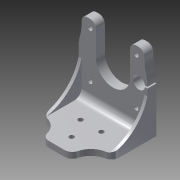
# Autodesk Inventor part: bottom-right bracket
Saved by Autodesk Inventor 2015 SP1 (Build 190203100, 203)
## iProperties
Created: 2015-01-03
Part Number: bottom-right bracket
Material: ABS Plastic
Document SubType Name: Modeling
Designer: Luna
Density: 1.06 g/cm^3
Appearance: Smooth - White
Mass: 2.06395 g
Surface Area: 14.6209 cm^2
Volume: 1.94712 cm^3
Author: Luna
Autodesk Inventor part; units mm, degrees
ref_plane "YZ Plane" through (0, 0, 0) normal (1, 0, 0) x (0, 1, 0)
ref_plane "XZ Plane" through (0, 0, 0) normal (0, 1, 0) x (-1, 0, 0)
ref_plane "XY Plane" through (0, 0, 0) normal (0, 0, 1) x (1, 0, 0)
sketch "hole points" plane through (0, 0, 0) normal (0, 0, 1) x (1, 0, 0)
  line L0 (-7, 0) -> (7, 0) construction
  line L1 (0, 0) -> (0, -13) construction
  dimension "d0" = 14
  dimension "d1" = 13
  constraints: 4 coincident, 4 end point, 1 horizontal, 1 midpoint, 1 vertical
  measures "d0" distance of L0.start L0.end
  measures "d1" distance of L1.start L1.end
sketch "Sketch3" plane through (0, 0, 0) normal (0, 0, 1) x (1, 0, 0)
  line L0 (-7, 0) -> (7, 0) construction
  line L1 (-7, 0) -> (7, 0) construction
  line L2 (-9, -2) -> (9, -2)
  line L3 (9, -2) -> (9, 2)
  line L4 (9, 2) -> (-9, 2)
  line L5 (-9, 2) -> (-9, -2)
  line L6 (-9, -2) -> (9, 2) construction
  line L7 (9, -2) -> (-9, 2) construction
  line L8 (0, 0) -> (0, -13) construction
  line L9 (-2, 2) -> (2, 2)
  line L10 (2, 2) -> (2, -15)
  line L11 (2, -15) -> (-2, -15)
  line L12 (-2, -15) -> (-2, 2)
  line L13 (17, -10) -> (-17, -10)
  line L14 (-17, -10) -> (-17, 10)
  line L15 (-17, 10) -> (17, 10)
  line L16 (17, 10) -> (17, -10)
  line L17 (10, -23) -> (10, 10)
  line L18 (10, 10) -> (-10, 10)
  line L19 (-10, 10) -> (-10, -23)
  line L20 (-10, -23) -> (10, -23)
  point P0 (0, -6.5)
  point P1 (0, 2)
  point P2 (0, -6.5)
  point P3 (0, 2)
  dimension "d31" = 18
  dimension "d32" = 4
  dimension "d33" = 4
  dimension "d34" = 17
  dimension "d35" = 8
  dimension "d36" = 8
  constraints: 40 end point, 8 parallel, 6 midpoint, 4 perpendicular, 2 horizontal, 1 coincident, 1 vertical alignment, 6 other
  measures "d31" distance of L4.end L3.end
  measures "d32" distance of L3.end L2.end
  measures "d33" distance of L10.end L11.end
  measures "d34" distance of L9.end L10.end
  measures "d35" distance between parallel lines of L2 L13
  measures "d36" distance between parallel lines of L10 L17
extrude "back plate Extrusion2" add sketch "Sketch3" against normal blind 4
hole "Hole3" at (-7, 0, 0) at (7, 0, 0) at (0, -13, 0) direction (0, 0, -1) diameter 3.2 end through all
sketch "Sketch4" plane through (-17, 10, 0) normal (0, 1, 0) x (1, 0, 0)
  circle A0 centre (17.85, -27.15) radius 11 projected
  circle A1 centre (2.35, -42.65) radius 1.5 projected
  circle A2 centre (33.35, -11.65) radius 1.5 projected
  circle A3 centre (33.35, -42.65) radius 1.5 projected
  circle A4 centre (2.35, -11.65) radius 1.5 projected
  line L0 (-3.3, -10) -> (0.7, -6) projected
  line L1 (-3.3, -44.3) -> (-3.3, -10) projected
  line L2 (0.7, -48.3) -> (-3.3, -44.3) projected
  line L3 (35, -48.3) -> (0.7, -48.3) projected
  line L4 (39, -44.3) -> (35, -48.3) projected
  line L5 (39, -10) -> (39, -44.3) projected
  line L6 (35, -6) -> (39, -10) projected
  line L7 (0.7, -6) -> (35, -6) projected
  line L8 (-3.3, 0) -> (39, 0)
  line L9 (39, 0) -> (39, 4)
  line L10 (39, 4) -> (-3.3, 4)
  line L11 (-3.3, 4) -> (-3.3, 0)
  line L12 (0, 4) -> (34, 4) projected
  point P0 (17, 0)
  point P1 (17.85, 4)
  point P2 (17, 4)
  point P3 (-3.3, 2)
  point P4 (39, 2)
  dimension "d44" = 4
  constraints: 8 end point, 4 midpoint, 2 parallel, 2 vertical alignment, 1 horizontal, 1 horizontal alignment, 1 perpendicular
  measures "d44" distance of L9.end L8.end
extrude "Extrusion3" add sketch "Sketch4" along normal blind 10 contours L11 L10 L9 L8
sketch "Sketch5" plane through (0, 0, 0) normal (0, 0, 1) x (1, 0, 0)
  line L0 (-16.3, 14) -> (18, 14) projected
  line L1 (-20.3, 20) -> (22, 20)
  line L2 (22, 20) -> (22, 14)
  line L3 (22, 14) -> (-20.3, 14)
  line L4 (-20.3, 14) -> (-20.3, 20)
  point P0 (0, 0)
  dimension "d47" = 42.3
  constraints: 8 end point, 2 parallel, 1 horizontal, 1 perpendicular, 1 point on line
  measures "d47" distance between parallel lines of L2 L4
extrude "Extrusion4" add sketch "Sketch5" along normal blind 48
sketch "Sketch6" plane through (-17, 20, 0) normal (0, 1, 0) x (1, 0, 0)
  circle A0 centre (17.85, -27.15) radius 10.5 projected
  circle A1 centre (17.85, -27.15) radius 11.5
  circle A2 centre (2.35, -42.65) radius 1.5 construction
  circle A3 centre (33.35, -42.65) radius 1.5 construction
  circle A4 centre (33.35, -11.65) radius 1.5 construction
  circle A5 centre (2.35, -11.65) radius 1.5 construction
  line L0 (6.35, -27.15) -> (6.35, -48)
  line L1 (39, -48) -> (-3.3, -48) projected
  line L2 (29.35, -27.15) -> (29.35, -48)
  line L3 (29.35, -48) -> (6.35, -48)
  point P0 (17, 0)
  dimension "d50" = 1
  constraints: 6 end point, 2 point on circle, 2 point on line, 2 tangent, 1 centre point, 1 collinear, 1 parallel, 1 vertical
  measures "d50" radial gap between concentric circles of A0 A1
extrude "Extrusion5" cut sketch "Sketch6" against normal through all contours A0 | A1 | L2 L1 L0 A1
sketch "Sketch7" plane through (-17, 20, 0) normal (0, 1, 0) x (1, 0, 0)
  circle A0 centre (2.35, -42.65) radius 1.5 projected
  circle A1 centre (33.35, -42.65) radius 1.5 projected
  circle A2 centre (33.35, -11.65) radius 1.5 projected
  circle A3 centre (2.35, -11.65) radius 1.5 projected
  point P0 (17, 0)
hole "Hole4" at (-14.65, 20, 11.65) at (16.35, 20, 11.65) at (16.35, 20, 42.65) at (-14.65, 20, 42.65) direction (0, -1, 0) diameter 3.2 end through all
sketch "Sketch8" plane through (22, 10, 0) normal (1, 0, 0) x (0, 0, -1)
  line L0 (-24.65, 27.5) -> (-29.65, 27.5) projected
  line L1 (-22.15, 4) -> (-32.15, 4)
  line L2 (-32.15, 4) -> (-32.15, 10)
  line L3 (-32.15, 10) -> (-22.15, 10)
  line L4 (-22.15, 10) -> (-22.15, 4)
  point P0 (0, -10)
  point P1 (-27.15, 10)
  point P2 (-27.15, 27.5)
  point P3 (-27.15, 10)
  dimension "d62" = 10
  dimension "d63" = 6
  constraints: 8 end point, 2 midpoint, 2 parallel, 1 coincident, 1 horizontal, 1 perpendicular, 1 vertical alignment
  measures "d62" distance of L2.end L3.end
  measures "d63" distance of L1.end L2.end
extrude "Extrusion6" add sketch "Sketch8" along normal blind 2
sketch "Sketch9" plane through (-17, 20, 0) normal (0, 1, 0) x (1, 0, 0)
  circle A0 centre (17.85, -27.15) radius 2.5 construction
  line L0 (17.85, -27.15) -> (35.35, -27.15) construction
  point P0 (17, 0)
  dimension "d66" = 17.5
  constraints: 2 end point, 1 horizontal
  measures "d66" distance of L0.start L0.end
hole "Hole5" at (18.35, 20, 27.15) direction (0, -1, 0) diameter 8 end through all
sketch "Sketch10" plane through (24, 10, 0) normal (1, 0, 0) x (0, 0, -1)
  line L0 (-32.15, 4) -> (-22.15, 4) projected
  line L1 (-22.15, 4) -> (-22.15, 10) projected
  line L2 (-22.15, 10) -> (-32.15, 10) projected
  line L3 (-32.15, 10) -> (-32.15, 4) projected
  line L4 (-27.65, 10) -> (-26.65, 10)
  line L5 (-26.65, 10) -> (-26.65, 4)
  line L6 (-26.65, 4) -> (-27.65, 4)
  line L7 (-27.65, 4) -> (-27.65, 10)
  line L8 (-22.15, 10) -> (-32.15, 10) projected
  point P0 (0, -10)
  point P1 (-27.15, 10)
  point P2 (-27.15, 10)
  point P3 (-27.15, 10)
  dimension "d74" = 1
  dimension "d75" = 6
  constraints: 8 end point, 3 midpoint, 2 coincident, 2 parallel, 1 horizontal, 1 perpendicular
  measures "d74" distance of L4.start L4.end
  measures "d75" distance of L4.end L5.end
extrude "Extrusion7" cut sketch "Sketch10" against normal blind 5 contours L7 L2 L5 L0
sketch "Sketch11" plane through (-17, -10, -4) normal (-1, 0, 0) x (0, 0, 1)
  line L0 (4, 0) -> (4, 20) projected
  line L1 (4, 20) -> (0, 20) projected
  line L2 (0, 0) -> (0, 20) projected
  line L3 (4, 0) -> (0, 0) projected
  point P0 (4, 10)
extrude "Extrusion8" add sketch "Sketch11" along normal blind 3.3
sketch "Sketch12" plane through (17, -10, 0) normal (1, 0, 0) x (0, 0, -1)
  line L0 (0, 20) -> (0, 0) projected
  line L1 (0, 0) -> (4, 0) projected
  line L2 (4, 20) -> (4, 0) projected
  line L3 (0, 20) -> (4, 20) projected
  point P0 (0, 10)
extrude "Extrusion9" add sketch "Sketch12" along normal blind 5
fillet "Fillet3" radius 4 4 edges at (22, 17, 48) (12.35, 17, 48) (-10.65, 17, 48) (-20.3, 17, 48)
fillet "Fillet6" radius 5 1 edges at (0.85, 14, 0)
sketch "Sketch15" plane through (22, -10, -4) normal (1, 0, 0) x (0, 0, -1)
  line L0 (-26.15, 30) -> (-26.15, 24) projected
  line L1 (-9, 24) -> (-26.15, 24) projected
  arc A0 (-4, 19) -> (-9, 24) centre (-9, 19) ccw projected
  line L2 (-4, 0) -> (-4, 19) projected
  line L3 (-4, 0) -> (0, 0) projected
  line L4 (0, 0) -> (0, 30) projected
  line L5 (0, 30) -> (-26.15, 30) projected
  arc A1 (-4, 0) -> (-26.15, 24) centre (-33.5688, -5.0682) ccw
  line L6 (-26.15, 24) -> (-26.15, 30)
  line L7 (-26.15, 30) -> (0, 30)
  line L8 (0, 30) -> (-26.15, 30) projected
  line L9 (0, 30) -> (0, 0)
  line L10 (0, 0) -> (0, 30) projected
  line L11 (0, 0) -> (-4, 0)
  point P0 (-4, 10)
  dimension "d97" = 30
  constraints: 8 end point, 4 collinear, 2 point on circle, 1 centre point
  measures "d97" radius of A1
extrude "Extrusion12" add sketch "Sketch15" along normal blind 2
sketch "Sketch16" plane through (-20.3, -10, -4) normal (-1, 0, 0) x (0, 0, 1)
  line L0 (30.65, 30) -> (30.65, 24) projected
  line L1 (30.65, 24) -> (26.15, 24) projected
  arc A0 (26.15, 24) -> (4, 0) centre (33.5688, -5.0682) ccw projected
  line L2 (4, 0) -> (0, 0) projected
  line L3 (0, 0) -> (0, 30) projected
  line L4 (0, 30) -> (30.65, 30) projected
  point P0 (4, 10)
extrude "Extrusion13" add sketch "Sketch16" along normal blind 2
fillet "Fillet10" radius 12 2 edges at (-10, -10, -2) (10, -10, -2)
fillet "Fillet11" radius 5 4 edges at (-22.3, -10, -2) (-10, -23, -2) (10, -23, -2) (24, -10, -2)
sketch "Sketch17" plane through (-20.3, 14, 26.65) normal (0, 0, 1) x (1, 0, 0)
  line L0 (0, 6) -> (0, 0) projected
  line L1 (0, 6) -> (-2, 6) projected
  line L2 (-2, 0) -> (-2, 6) projected
  line L3 (0, 0) -> (-2, 0) projected
  point P0 (20.3, -14)
extrude "Extrusion14" add sketch "Sketch17" along normal blind 5.5
fillet "Fillet14" radius 25 2 edges at (-20.3, 17, 32.15) (22, 17, 32.15)
fillet "Fillet15" radius 20 2 edges at (-22.3, 17, 32.15) (24, 17, 32.15)
body "Solid2"
